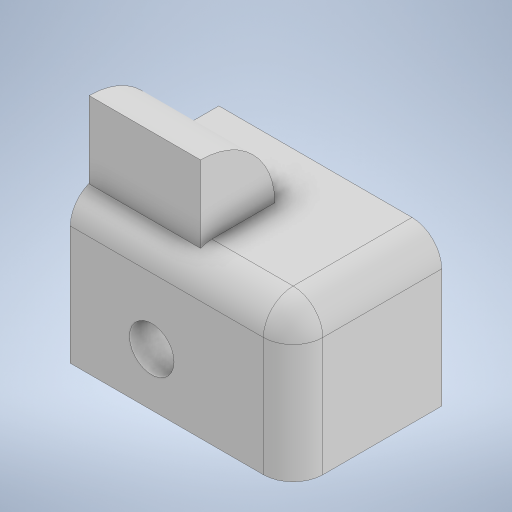
# Autodesk Inventor part: TEAM4788-001-Test-Part
Saved by Autodesk Inventor 2023.2 (Build 272271000, 271)
## iProperties
Created: 2023-10-07
Part Number: TEAM4788-001-Test-Part
Material: Generic
Document SubType Name: Modeling
Designer: 271663e
Density: 1 g/cm^3
Appearance: Default
Author: 271663e
Autodesk Inventor part; units mm, degrees
ref_plane "YZ Plane" through (0, 0, 0) normal (1, 0, 0) x (0, 1, 0)
ref_plane "XZ Plane" through (0, 0, 0) normal (0, 1, 0) x (-1, 0, 0)
ref_plane "XY Plane" through (0, 0, 0) normal (0, 0, 1) x (1, 0, 0)
sketch "Sketch1" plane through (0, 0, 0) normal (0, 1, 0) x (-1, 0, 0)
  line L0 (0, 0) -> (-15, 0)
  line L1 (-15, 0) -> (-15, -10)
  line L2 (-15, -10) -> (0, -10)
  line L3 (0, -10) -> (0, 0)
  dimension "d0" = 10
  dimension "d1" = 15
  constraints: 8 end point, 2 parallel, 1 horizontal, 1 perpendicular
  measures "d0" distance of L0.end L1.end
  measures "d1" distance of L1.end L2.end
extrude "Extrusion1" add sketch "Sketch1" along normal blind 10
sketch "Sketch2" plane through (0, 10, 0) normal (0, 1, 0) x (1, 0, 0)
  line L0 (0.0305, 1.2348) -> (7.5305, 1.2348)
  line L1 (7.5305, 1.2348) -> (7.5305, 6.2348)
  line L2 (7.5305, 6.2348) -> (0.0305, 6.2348)
  line L3 (0.0305, 6.2348) -> (0.0305, 1.2348)
  point P0 (0, 0)
  dimension "d4" = 5
  dimension "d5" = 7.5
  constraints: 8 end point, 2 parallel, 1 horizontal, 1 perpendicular
  measures "d4" distance of L0.end L1.end
  measures "d5" distance of L1.end L2.end
revolve "Revolution1" add sketch "Sketch2" angle 90 about axis through (0.0305, 10, -1.2348) along (1, 0, 0)
fillet "Fillet1" radius 2 3 edges at (7.5, 10, 0) (15, 10, -5) (15, 5, 0)
sketch "Sketch3" plane through (0, 0, 0) normal (0, 0, 1) x (1, 0, 0)
  point P0 (0, 0)
  point P1 (5.4835, 3.5664)
hole "Hole1" at (5.4835, 3.5664, 0) direction (0, 0, -1) diameter 3 end through all
body "Solid1"
